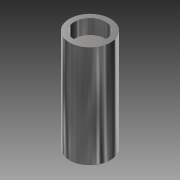
# Autodesk Inventor part: Shaft
Saved by Autodesk Inventor 2014 SP2 (Build 180246200, 246)
## iProperties
Created: 2019-06-15
Part Number: Shaft
Material: Generic
Document SubType Name: Modeling
Designer: Yuchofif
Density: 1 g/cm^3
Appearance: Default
Author: Yuchofif
Autodesk Inventor part; units mm, degrees
ref_plane "YZ Plane" through (0, 0, 0) normal (1, 0, 0) x (0, 1, 0)
ref_plane "XY Plane" through (0, 0, 0) normal (0, 0, 1) x (1, 0, 0)
sketch "Sketch1" plane through (0, 0, 0) normal (0, 0, 1) x (1, 0, 0)
  circle A0 centre (0, 0) radius 7
  constraints: 1 centre point, 1 coincident
extrude "Extrusion1" add sketch "Sketch1" against normal blind 35
sketch "Sketch2" plane through (0, 0, 0) normal (0, 0, 1) x (1, 0, 0)
  circle A0 centre (0, 0) radius 7 projected
  circle A1 centre (0, 0) radius 5.25
  constraints: 1 centre point, 1 coincident
extrude "Extrusion2" cut sketch "Sketch2" against normal blind 5 contours A1
sketch "Sketch3" plane through (0, 0, -5) normal (0, 0, 1) x (1, 0, 0)
  circle A0 centre (0, 0) radius 5.25 projected
  circle A1 centre (0, 0) radius 1.5
  constraints: 1 centre point, 1 coincident
extrude "Extrusion3" cut sketch "Sketch3" against normal blind 30 contours A1
sketch "Sketch4" plane through (0, 0, -35) normal (0, 0, -1) x (-1, 0, 0)
  circle A0 centre (0, 0) radius 1.5 projected
  circle A1 centre (0, 0) radius 7 projected
  circle A2 centre (0, 0) radius 1.5
  circle A3 centre (0, 0) radius 3
  constraints: 2 centre point, 2 coincident, 1 concentric
extrude "Extrusion4" cut sketch "Sketch4" against normal blind 9 contours A3
ref_plane "Work Plane1" through (0, 9, 0) normal (0, 1, 0) x (-1, 0, 0)
sketch "Sketch5" plane through (0, 9, 0) normal (0, 1, 0) x (-1, 0, 0)
  line L0 (3, -35) -> (-3, -35) projected
  line L1 (-7, -35) -> (7, -35) projected
  circle A0 centre (0, -29) radius 1.5
  point P0 (0, 0)
  constraints: 1 centre point
extrude "Extrusion5" cut sketch "Sketch5" against normal blind 9
thread "Thread1" size "M3x0.5" class "6H" standard "ANSI Metric M Profile" full length
fillet "Fillet1" radius 0.4 1 edges at (-7, 0, -35)
body "Solid1"
